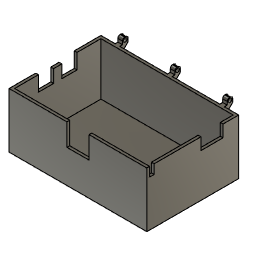
桶身 (Autodesk Fusion 360 design; units mm, degrees)
part number: 2025-05-27-14-06-25-822
Autodesk Fusion 360 part; units mm, degrees
sketch "草图1" plane through (75, 0, 0) normal (1, 0, 0) x (0, 1, 0)
  line L0 (100, 100) -> (103, 100)
  line L1 (103, 100) -> (103, 103.5)
  line L2 (105.5, 106) -> (106.5, 106)
  line L3 (109, 103.5) -> (109, 100)
  line L4 (108.7423, 99.3777) -> (100, 90.6355)
  circle A0 centre (106, 103) radius 2
  line L5 (100, 0) -> (100, 100)
  arc A1 (105.5, 106) -> (103, 103.5) centre (105.5, 103.5) ccw
  arc A2 (109, 103.5) -> (106.5, 106) centre (106.5, 103.5) ccw
  arc A3 (108.7423, 99.3777) -> (109, 100) centre (108.12, 100) ccw
  point P0 (100, 100)
  dimension "d1" = 3
  dimension "d2" = 4
  dimension "d3" = 3
  dimension "d6" = 3
  dimension "d9" = 3
  dimension "d10" = 3
  dimension "d13" = 135
  dimension "d14" = 2.5
  dimension "d15" = 2.5
  dimension "d16" = 0.88
  constraint horizontal L0
  constraint perpendicular L0 L1
  constraint perpendicular L1 L2
  constraint perpendicular L2 L3
  constraint coincident P0 L0.start
  constraint coincident L4.end L5
  constraint tangent L2 A1
  constraint tangent L1 A1
  constraint tangent L2 A2
  constraint tangent L3 A2
  constraint tangent L3 A3
  constraint tangent L4 A3
  constraint equal L1 L3
  measures "d1" distance of P0 L0.end
  measures "d2" diameter of A0
  measures "d3" distance of L1 A0.centre
  measures "d6" distance of L3 A0.centre
  measures "d9" distance of L2 A0.centre
  measures "d10" vertical distance of L0.end A0.centre
  measures "d13" angle of L3 L4
  measures "d14" radius of A1
  measures "d15" radius of A2
  measures "d16" radius of A3
sketch "草图2" plane through (18, 0, 0) normal (1, 0, 0) x (0, 1, 0)
  arc A0 (108.7423, 99.3777) -> (109, 100) centre (108.12, 100) ccw
  arc A1 (105.5, 106) -> (103, 103.5) centre (105.5, 103.5) ccw
  line L0 (105.5, 106) -> (106.5, 106)
  line L1 (100, 100) -> (103, 100)
  arc A2 (109, 103.5) -> (106.5, 106) centre (106.5, 103.5) ccw
  circle A3 centre (106, 103) radius 2
  line L2 (109, 103.5) -> (109, 100)
  line L3 (108.7423, 99.3777) -> (100, 90.6355)
  line L4 (103, 100) -> (103, 103.5)
  line L5 (100, 0) -> (100, 100)
  point P0 (100, 100)
  point P1 (100, 100)
  point P2 (100, 100)
  dimension "d17" = 3
  dimension "d18" = 4
  dimension "d21" = 3
  dimension "d22" = 3
  dimension "d23" = 3
  dimension "d26" = 3
  dimension "d27" = 135
  dimension "d30" = 2.5
  dimension "d31" = 2.5
  dimension "d32" = 0.88
  constraint horizontal L1
  constraint perpendicular L1 L4
  constraint perpendicular L0 L4
  constraint perpendicular L0 L2
  constraint coincident P2 P1
  constraint tangent A1 L0
  constraint tangent A1 L4
  constraint tangent L0 A2
  constraint tangent A2 L2
  constraint tangent A0 L2
  constraint tangent A0 L3
  constraint equal L2 L4
  constraint coincident L3.end L5
  measures "d17" distance of L1.end P2
  measures "d18" diameter of A3
  measures "d21" distance of A3.centre L4
  measures "d22" distance of A3.centre L2
  measures "d23" distance of A3.centre L0
  measures "d26" vertical distance of L1.end A3.centre
  measures "d27" angle of L2 L3
  measures "d30" radius of A1
  measures "d31" radius of A2
  measures "d32" radius of A0
sketch "草图3" plane through (147, 0, 0) normal (-1, 0, 0) x (0, -1, 0)
  line L0 (-59, 100) -> (-59, 87)
  line L1 (-59, 87) -> (-83, 87)
  line L2 (-83, 87) -> (-83, 100)
  line L3 (-83, 100) -> (-97, 100)
  line L4 (-97, 100) -> (-97, 3)
  line L5 (-97, 3) -> (-3, 3)
  line L6 (-3, 3) -> (-3, 100)
  line L7 (-3, 100) -> (-59, 100)
  line L8 (-8, 100) -> (-3, 100)
  line L9 (-3, 100) -> (-3, 90)
  line L10 (-3, 90) -> (-8, 90)
  line L11 (-8, 90) -> (-8, 100)
  dimension "d33" = 5
  dimension "d34" = 10
  constraint horizontal L8
  constraint vertical L9
  constraint horizontal L10
  constraint vertical L11
  constraint coincident L7 L8.start
  constraint collinear L6 L9
  measures "d33" distance of L8.start L6.end
  measures "d34" distance of L8.start L10.end
sketch "草图4" plane through (132, 0, 0) normal (-1, 0, 0) x (0, -1, 0)
  line L0 (-100, 100) -> (-103, 100)
  line L1 (-105.5, 106) -> (-106.5, 106)
  arc A0 (-106.5, 106) -> (-109, 103.5) centre (-106.5, 103.5) ccw
  line L2 (-103, 100) -> (-103, 103.5)
  arc A1 (-103, 103.5) -> (-105.5, 106) centre (-105.5, 103.5) ccw
  circle A2 centre (-106, 103) radius 2
  line L3 (-109, 103.5) -> (-109, 100)
  arc A3 (-109, 100) -> (-108.7657, 99.4343) centre (-108.2, 100) ccw
  line L4 (-108.7657, 99.4343) -> (-100, 90.6686)
  line L5 (-100, 0) -> (-100, 100)
  point P0 (-105.9337, 94.2405)
  point P1 (-105.9337, 94.2405)
  point P2 (-100, 100)
  dimension "d35" = 3.5
  dimension "d36" = 3
  dimension "d37" = 3
  dimension "d38" = 3
  dimension "d39" = 3
  dimension "d42" = 3
  dimension "d43" = 1
  dimension "d44" = 4
  dimension "d45" = 0.8
  dimension "d46" = 135
  constraint equal L2 L3
  constraint horizontal L1
  constraint vertical L2
  constraint tangent L1 A1
  constraint tangent L1 A0
  constraint tangent L2 A1
  constraint tangent A0 L3
  constraint tangent L3 A3
  constraint tangent A3 L4
  constraint perpendicular L0 L2
  constraint coincident P2 L0.start
  constraint coincident L4.end L5
  constraint vertical L3
  measures "d35" distance of L0.end L2.end
  measures "d36" distance of P2 L0.end
  measures "d37" distance of A2.centre L2
  measures "d38" distance of A2.centre L1
  measures "d39" distance of A2.centre L3
  measures "d42" vertical distance of L0.end A2.centre
  measures "d43" distance of L1.start L1.end
  measures "d44" diameter of A2
  measures "d45" radius of A3
  measures "d46" angle of L3 L4
sketch "草图5" plane through (0, 0, 0) normal (0, -1, 0) x (1, 0, 0)
  line L0 (0, 0) -> (150, 0)
  line L1 (150, 0) -> (150, 100)
  line L2 (150, 100) -> (0, 100)
  line L3 (0, 100) -> (0, 0)
  line L4 (63, 100) -> (87, 100)
  line L5 (87, 100) -> (87, 76)
  line L6 (87, 76) -> (63, 76)
  line L7 (63, 76) -> (63, 100)
  dimension "d47" = 24
  dimension "d48" = 24
  constraint horizontal L4
  constraint vertical L5
  constraint horizontal L6
  constraint vertical L7
  constraint midpoint L2 L4
  measures "d47" distance of L4.start L4.end
  measures "d48" distance of L4.start L6.end
sketch "草图6" plane through (0, 0, 0) normal (-1, 0, 0) x (0, -1, 0)
  line L0 (-100, 0) -> (0, 0)
  line L1 (0, 0) -> (0, 100)
  line L2 (0, 100) -> (-100, 100)
  line L3 (-100, 100) -> (-100, 0)
  line L4 (-71, 100) -> (-54.5, 100)
  line L5 (-54.5, 100) -> (-54.5, 83.5)
  line L6 (-54.5, 83.5) -> (-71, 83.5)
  line L7 (-71, 83.5) -> (-71, 100)
  line L8 (-45.5, 100) -> (-29, 100)
  line L9 (-29, 100) -> (-29, 83.5)
  line L10 (-29, 83.5) -> (-45.5, 83.5)
  line L11 (-45.5, 83.5) -> (-45.5, 100)
  line L12 (-54.5, 100) -> (-45.5, 100) construction
  line L13 (-54.5, 100) -> (-45.5, 100)
  line L14 (-45.5, 100) -> (-45.5, 97.5)
  line L15 (-45.5, 97.5) -> (-54.5, 97.5)
  line L16 (-54.5, 97.5) -> (-54.5, 100)
  dimension "d49" = 16.5
  dimension "d50" = 16.5
  dimension "d51" = 16.5
  dimension "d52" = 16.5
  dimension "d53" = 9
  dimension "d56" = 14
  constraint horizontal L4
  constraint vertical L5
  constraint horizontal L6
  constraint vertical L7
  constraint horizontal L8
  constraint vertical L9
  constraint horizontal L10
  constraint vertical L11
  constraint collinear L4 L8
  constraint midpoint L2 L12
  constraint horizontal L13
  constraint vertical L14
  constraint horizontal L15
  constraint vertical L16
  constraint coincident L11 L14.end
  measures "d49" distance of L4.start L4.end
  measures "d50" distance of L4.start L6.end
  measures "d51" distance of L8.start L8.end
  measures "d52" distance of L8.start L10.end
  measures "d53" distance of L5 L11
  measures "d56" distance of L6 L15
sketch "草图7" plane through (0, 0, 3) normal (0, 0, 1) x (-1, 0, 0)
  line L0 (0, -100) -> (0, 0)
  line L1 (0, 0) -> (-150, 0)
  line L2 (-150, 0) -> (-150, -100)
  line L3 (-150, -100) -> (0, -100)
  line L4 (-3, -3) -> (-147, -3)
  line L5 (-147, -3) -> (-147, -97)
  line L6 (-147, -97) -> (-3, -97)
  line L7 (-3, -97) -> (-3, -3)
  dimension "d57" = -3
sketch "草图8" plane through (150, 0, 0) normal (1, 0, 0) x (0, 1, 0)
  line L0 (0, 0) -> (100, 0)
  line L1 (100, 0) -> (100, 100)
  line L2 (100, 100) -> (0, 100)
  line L3 (0, 100) -> (0, 0)
  line L4 (59, 100) -> (83, 100)
  line L5 (83, 100) -> (83, 87)
  line L6 (83, 87) -> (59, 87)
  line L7 (59, 87) -> (59, 100)
  dimension "d58" = 24
  dimension "d59" = 13
  dimension "d60" = 17
  constraint horizontal L4
  constraint vertical L5
  constraint horizontal L6
  constraint vertical L7
  constraint coincident L2 L4.start
  measures "d58" distance of L4.start L4.end
  measures "d59" distance of L4.start L6.end
  measures "d60" distance of L1 L5
sketch "草图9" plane through (0, 0, 0) normal (0, 0, 1) x (1, 0, 0)
  line L0 (0, 0) -> (150, 0)
  line L1 (150, 0) -> (150, 100)
  line L2 (150, 100) -> (0, 100)
  line L3 (0, 100) -> (0, 0)
  dimension "d61" = 150
  dimension "d62" = 100
  constraint horizontal L0
  constraint vertical L1
  constraint horizontal L2
  constraint vertical L3
  constraint coincident L0.start L3.end
  measures "d61" distance of L0.start L0.end
  measures "d62" distance of L0.start L2.end
extrude "拉伸1" add sketch "草图9" along normal blind 3
extrude "拉伸2" add sketch "草图7" along normal blind 97
extrude "拉伸3" cut sketch "草图5" against normal blind 25 contours L2 L4 L5 L6 L7
extrude "拉伸4" cut sketch "草图6" against normal blind 10 contours L2 L4 L5 L6 L7 L16 | L2 L8 L9 L10 L11 L14 | L2 L5 L11 L13 L14 L15 L16
extrude "拉伸5" cut sketch "草图8" against normal blind 20 contours L2 L4 L5 L6 L7
extrude "拉伸6" cut sketch "草图3" against normal blind 10 contours L6 L7 L8 L9 L10 L11
extrude "拉伸7" add sketch "草图1" along normal mid plane 5
extrude "拉伸8" add sketch "草图2" along normal mid plane 5
extrude "拉伸9" add sketch "草图4" along normal mid plane 5
extrude "拉伸10" add 1 faces at (51, 65.6667, 3) along direction (0, 0, 1) blind 40
extrude "拉伸11" cut 1 faces at (50, 66.6667, 0) along direction (0, 0, 1) blind 40
equation "d7 = 100 mm - 3 mm"
